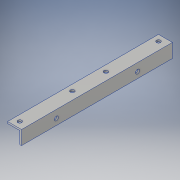
# Autodesk Inventor part: bepf_platforma_rama_bok_krotki
Saved by Autodesk Inventor 2017 (Build 210142000, 142)
## iProperties
Created: 2016-11-24
Part Number: bepf_platforma_rama_bok_krotki
Material: Aluminium 6061
Document SubType Name: Modeling
Designer: gagato
Density: 2.7 g/cm^3
Appearance: Aluminium — płaski
Mass: 11.6125 g
Surface Area: 62.9101 cm^2
Volume: 4.30091 cm^3
Author: gagato
Autodesk Inventor part; units mm, degrees
ref_plane "YZ Plane" through (0, 0, 0) normal (1, 0, 0) x (0, 1, 0)
ref_plane "XZ Plane" through (0, 0, 0) normal (0, 1, 0) x (-1, 0, 0)
ref_plane "XY Plane" through (0, 0, 0) normal (0, 0, 1) x (1, 0, 0)
sketch "Szkic1" plane through (0, 0, 0) normal (0, 0, 1) x (1, 0, 0)
  line L0 (0, 0) -> (0, 12)
  line L1 (0, 12) -> (-1.5, 12)
  line L2 (-1.5, 12) -> (-1.5, 1.5)
  line L3 (-1.5, 1.5) -> (-12, 1.5)
  line L4 (-12, 1.5) -> (-12, 0)
  line L5 (-12, 0) -> (0, 0)
  dimension "d0" = 12
  dimension "d1" = 1.5
  dimension "d2" = 10.5
  dimension "d3" = 10.5
  constraints: 12 end point, 5 perpendicular, 1 vertical
  measures "d0" distance of L0.start L0.end
  measures "d1" distance of L0.end L1.end
  measures "d2" distance of L1.end L2.end
  measures "d3" distance of L2.end L3.end
extrude "Wyciągnięcie proste1" add sketch "Szkic1" along normal mid plane 130
move or copy body "Przesuń bryłę1" bodies to move or copy 1 copy no rotation origin (0, 0, 0) rotation axis (0, 0, 1) rotation angle 90
sketch "Szkic2" plane through (-12, 0, 65) normal (0, 1, 0) x (1, 0, 0)
  line L0 (12, 0) -> (0, 0) projected
  line L1 (12, 0) -> (12, 130) projected
  line L2 (0, 130) -> (0, 0) construction
  line L3 (0, 65) -> (5.25, 65) construction
  line L4 (5.25, 79.5) -> (5.25, 50.5) construction
  point P0 (12, 65)
  dimension "d16" = 5.25
  dimension "d17" = 29
  constraints: 4 end point, 2 coincident, 2 midpoint, 1 horizontal, 1 vertical
  measures "d16" distance of L3.end L3.start
  measures "d17" distance of L4.start L4.end
hole "Otwór1" at (-6.75, 0, -14.5) at (-6.75, 0, 14.5) direction (0, -1, 0) diameter 3.5 end through all
sketch "Szkic3" plane through (-12, 0, 65) normal (0, 1, 0) x (1, 0, 0)
  line L0 (0, 130) -> (0, 0) construction
  line L1 (12, 0) -> (0, 0) construction
  point P0 (12, 65)
  point P1 (5.25, 5.25)
  dimension "d19" = 5.25
  dimension "d20" = 5.25
  measures "d19" distance from line of L1 point (5.25, 5.25)
  measures "d20" distance from line of L0 point (5.25, 5.25)
hole "Otwór2" at (-6.75, 0, 59.75) direction (0, -1, 0) diameter 3.5 end through all
mirror "Odbij1" about plane through (0, 0, 0) normal (0, 0, 1) of "Otwór2"
sketch "Szkic5" plane through (0, -12, 65) normal (1, 0, 0) x (0, 0, -1)
  line L0 (130, 0) -> (0, 0) construction
  line L1 (65, 0) -> (65, 5.25) construction
  line L2 (30, 5.25) -> (100, 5.25) construction
  point P0 (65, 12)
  dimension "d37" = 5.25
  dimension "d38" = 70
  constraints: 4 end point, 2 coincident, 2 midpoint, 1 horizontal, 1 vertical
  measures "d37" distance of L1.end L1.start
  measures "d38" distance of L2.start L2.end
hole "Otwór4" at (0, -6.75, 35) at (0, -6.75, -35) direction (-1, 0, 0) diameter 3.5 end through all
